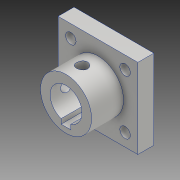
# Autodesk Inventor part: 1225a_Pinion Collar_V1
Saved by Autodesk Inventor 2020 (Build 240168000, 168)
## iProperties
Created: 2019-09-12
Part Number: 1225a_Pinion Collar_V1
Material: Aluminum 6061
Document SubType Name: Modeling
Designer: MPI
Density: 2.7 g/cm^3
Appearance: Aluminum - Flat
Author: MPI
Autodesk Inventor part; units mm, degrees
ref_plane "YZ Plane" through (0, 0, 0) normal (1, 0, 0) x (0, 1, 0)
ref_plane "XZ Plane" through (0, 0, 0) normal (0, 1, 0) x (-1, 0, 0)
ref_plane "XY Plane" through (0, 0, 0) normal (0, 0, 1) x (1, 0, 0)
sketch "Sketch1" plane through (0, 0, 0) normal (0, 1, 0) x (-1, 0, 0)
  circle A0 centre (0, 0) radius 10
  circle A1 centre (0, 0) radius 16
  dimension "d0" = 20
  dimension "d1" = 32
  constraints: 2 centre point, 2 coincident
  measures "d0" diameter of A0
  measures "d1" diameter of A1
extrude "Extrusion1" add sketch "Sketch1" along normal blind 30
sketch "Sketch4" plane through (0, 0, 0) normal (0, 0, 1) x (1, 0, 0)
  circle A0 centre (0, 10) radius 3.45
  line L0 (-16, 0) -> (16, 0) projected
  point P0 (0, 0)
  dimension "d13" = 6.9
  dimension "d14" = 10
  constraints: 1 centre point
  measures "d13" diameter of A0
  measures "d14" distance from line of L0 A0.centre
extrude "Extrusion4" cut sketch "Sketch4" along normal blind 30
sketch "Sketch5" plane through (0, 0, 0) normal (1, 0, 0) x (0, 1, 0)
  circle A0 centre (10, 0) radius 3.45
  line L0 (0, 16) -> (0, -16) projected
  point P0 (0, 0)
  dimension "d17" = 6.9
  dimension "d18" = 10
  constraints: 1 centre point
  measures "d17" diameter of A0
  measures "d18" distance from line of L0 A0.centre
extrude "Extrusion5" cut sketch "Sketch5" against normal blind 30
sketch "Sketch6" plane through (0, 0, 0) normal (0, -1, 0) x (1, 0, 0)
  line L0 (-3.05, -9.5235) -> (3.05, -9.5235)
  line L1 (3.05, -9.5235) -> (3.05, -12.5735)
  line L2 (3.05, -12.5735) -> (-3.05, -12.5735)
  line L3 (-3.05, -12.5735) -> (-3.05, -9.5235)
  circle A0 centre (0, 0) radius 10 projected
  dimension "d21" = 6.1
  dimension "d22" = 3.05
  constraints: 8 end point, 2 parallel, 2 point on circle, 1 horizontal, 1 perpendicular
  measures "d21" distance of L1.end L2.end
  measures "d22" distance of L0.end L1.end
extrude "Extrusion6" cut sketch "Sketch6" against normal through all contours A0 L1 L2 L3 | L0 A0 picked at (0.3438, -9.6646)
sketch "Sketch9" plane through (0, 30, 0) normal (0, 1, 0) x (1, 0, 0)
  line L0 (-25, -25) -> (25, -25)
  line L1 (25, -25) -> (25, 25)
  line L2 (25, 25) -> (-25, 25)
  line L3 (-25, 25) -> (-25, -25)
  circle A0 centre (-17, -17) radius 3.265
  circle A1 centre (-17, 17) radius 3.265
  circle A2 centre (17, -17) radius 3.265
  circle A3 centre (17, 17) radius 3.265
  circle A4 centre (0, 0) radius 16
  dimension "d25" = 50
  dimension "d26" = 50
  dimension "d27" = 25
  dimension "d28" = 25
  dimension "d29" = 6.53
  dimension "d30" = 8
  dimension "d31" = 8
  dimension "d32" = 8
  dimension "d33" = 8
  dimension "d35" = 8
  dimension "d36" = 8
  dimension "d37" = 8
  dimension "d38" = 8
  constraints: 8 end point, 5 centre point, 3 equal radius, 2 parallel, 1 coincident, 1 horizontal, 1 perpendicular
  measures "d25" distance of L2.end L0.start
  measures "d26" distance of L1.end L2.end
  measures "d27" distance from line of point (0, 0) L3
  measures "d28" distance from line of point (0, 0) L2
  measures "d29" diameter of A0
  measures "d30" distance from line of L3 A0.centre
  measures "d31" distance from line of A0.centre L0
  measures "d32" distance from line of L2 A1.centre
  measures "d33" distance from line of A1.centre L3
  measures "d35" distance from line of L1 A3.centre
  measures "d36" distance from line of L2 A3.centre
  measures "d37" distance from line of L1 A2.centre
  measures "d38" distance from line of L0 A2.centre
extrude "Extrusion7" add sketch "Sketch9" against normal blind 10
body "Solid1"
